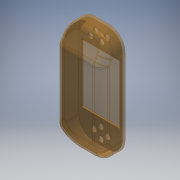
# Autodesk Inventor part: Dessous
Saved by Autodesk Inventor 2016 SP1 (Build 200210100, 210)
## iProperties
Created: 2018-06-04
Part Number: Dessous
Material: Polycarbonate, fumée
Document SubType Name: Modeling
Designer: dimercur
Mass: 856.8 g
Surface Area: 579.4 cm^2
Volume: 714 cm^3
Density: 1.2 g/cm^3
Appearance: Polycarbonate - Fumé
Author: dimercur
Autodesk Inventor part; units mm, degrees
ref_plane "YZ Plane" through (0, 0, 0) normal (1, 0, 0) x (0, 1, 0)
ref_plane "XZ Plane" through (0, 0, 0) normal (0, 1, 0) x (-1, 0, 0)
ref_plane "XY Plane" through (0, 0, 0) normal (0, 0, 1) x (1, 0, 0)
sketch "Esquisse1" plane through (0, 0, 0) normal (0, 1, 0) x (-1, 0, 0)
  line L0 (42.5, 100) -> (-42.5, 100)
  line L1 (-42.5, 100) -> (-42.5, -100)
  line L2 (-42.5, -100) -> (42.5, -100)
  line L3 (42.5, -100) -> (42.5, 100)
  point P0 (0, 0)
  dimension "d0" = 200
  dimension "d1" = 85
  dimension "d2" = 42.5
  dimension "d3" = 100
  constraints: 8 end point, 2 parallel, 1 horizontal, 1 perpendicular
  measures "d0" distance of L2.end L0.start
  measures "d1" distance of L0.start L0.end
  measures "d2" horizontal distance of point (0, 0) L0.start
  measures "d3" vertical distance of point (0, 0) L0.start
extrude "Extrusion1" add sketch "Esquisse1" along normal blind 42
chamfer "Chanfrein1" distance 20 angle 60 1 edges at (0, 0, 100) measured on face at (-14.1667, 14, 100)
chamfer "Chanfrein2" distance 20 angle 60 1 edges at (0, 0, -100) measured on face at (14.1667, 14, -100)
fillet "Congé3" radius 30 4 edges at (-42.5, 31, 100) (42.5, 31, 100) (-42.5, 31, -100) (42.5, 31, -100)
fillet "Congé4" radius 15 14 edges at (0, 0, 65.359) (-33.7132, 14.9269, 91.2132) (-42.5, 1.3397, 67.6795) (33.7132, 14.9269, 91.2132) (42.5, 1.3397, 67.6795) (0, 20, 100) (-42.5, 0, 0) (42.5, 0, 0) (0, 0, -65.359) (33.7132, 14.9269, -91.2132) (42.5, 1.3397, -67.6795) (-33.7132, 14.9269, -91.2132) (-42.5, 1.3397, -67.6795) (0, 20, -100)
shell "Coque1" thickness 2.5 removed faces 1 at (-14.1667, 42, -23.3333)
sketch "Esquisse3" plane through (0, 42, 0) normal (0, 1, 0) x (1, 0, 0)
  arc A0 (42.5, 70) -> (12.5, 100) centre (12.5, 70) ccw projected
  line L0 (12.5, 100) -> (-12.5, 100) projected
  arc A1 (-12.5, 100) -> (-42.5, 70) centre (-12.5, 70) ccw projected
  line L1 (-42.5, 70) -> (-42.5, -70) projected
  arc A2 (-42.5, -70) -> (-12.5, -100) centre (-12.5, -70) ccw projected
  line L2 (-12.5, -100) -> (12.5, -100) projected
  arc A3 (12.5, -100) -> (42.5, -70) centre (12.5, -70) ccw projected
  line L3 (42.5, -70) -> (42.5, 70) projected
  point P0 (0, 0)
extrude "Extrusion2" add sketch "Esquisse3" along normal blind 2.5
sketch "Esquisse4" plane through (0, 44.5, 0) normal (0, 1, 0) x (1, 0, 0)
  line L0 (35, 54) -> (-35, 54)
  line L1 (-35, 54) -> (-35, -54)
  line L2 (-35, -54) -> (35, -54)
  line L3 (35, -54) -> (35, 54)
  line L4 (27.5, -67.5897) -> (-27.5, -67.5897) projected
  circle A0 centre (-18.5, -67.5897) radius 5
  circle A1 centre (-8.5, -80) radius 5
  circle A2 centre (1.5, -67.5897) radius 5
  circle A3 centre (11.5, -80) radius 5
  circle A4 centre (12.5, 78) radius 5
  circle A5 centre (-12.5, 78) radius 5
  circle A6 centre (0.5, 88) radius 5
  circle A7 centre (0.5, 68) radius 5
  line L5 (42.5, -70) -> (42.5, 70) projected
  line L6 (-42.5, 70) -> (-42.5, -70) projected
  line L7 (12.5, 100) -> (-12.5, 100) projected
  line L8 (-12.5, -100) -> (12.5, -100) projected
  point P0 (0, 0)
  dimension "d19" = 108
  dimension "d20" = 70
  dimension "d21" = 35
  dimension "d22" = 54
  dimension "d23" = 10
  dimension "d24" = 10
  dimension "d25" = 10
  dimension "d26" = 10
  dimension "d27" = 10
  dimension "d28" = 10
  dimension "d29" = 10
  dimension "d30" = 10
  dimension "d31" = 25
  dimension "d32" = 12.5
  dimension "d33" = 20
  dimension "d34" = 42
  dimension "d35" = 42
  dimension "d36" = 30
  dimension "d37" = 22
  dimension "d38" = 24
  dimension "d39" = 20
  dimension "d40" = 20
  dimension "d41" = 20
  dimension "d42" = 20
  dimension "d43" = 34
  dimension "d44" = 12
  constraints: 8 centre point, 8 end point, 2 parallel, 2 point on line, 1 horizontal, 1 perpendicular
  measures "d19" distance of L2.end L0.start
  measures "d20" distance of L0.start L0.end
  measures "d21" horizontal distance of point (0, 0) L0.start
  measures "d22" vertical distance of point (0, 0) L0.start
  measures "d23" diameter of A6
  measures "d24" diameter of A4
  measures "d25" diameter of A7
  measures "d26" diameter of A5
  measures "d27" diameter of A2
  measures "d28" diameter of A3
  measures "d29" diameter of A1
  measures "d30" diameter of A0
  measures "d31" distance of A5.centre A4.centre
  measures "d32" horizontal distance of point (0, 0) A4.centre
  measures "d33" distance of A7.centre A6.centre
  measures "d34" distance from line of L5 A6.centre
  measures "d35" distance from line of L5 A7.centre
  measures "d36" distance from line of L6 A5.centre
  measures "d37" distance from line of L7 A4.centre
  measures "d38" distance from line of L6 A0.centre
  measures "d39" distance of A0.centre A2.centre
  measures "d40" distance of A3.centre A1.centre
  measures "d41" distance from line of L8 A1.centre
  measures "d42" distance from line of L8 A3.centre
  measures "d43" distance from line of L6 A1.centre
  measures "d44" distance from line of L7 A6.centre
extrude "Extrusion3" cut sketch "Esquisse4" against normal blind 3
equation "\"d2\" = 0.5 * d1"
equation "\"d3\" = 0.5 * d0"
equation "\"d21\" = 0.5 * d20"
equation "\"d22\" = 0.5 * d19"
equation "\"d32\" = 0.5 * d31"
